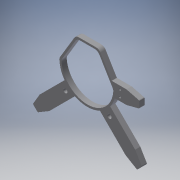
# Autodesk Inventor part: PearHeadbar
Saved by Autodesk Inventor 2016 (Build 200138000, 138)
## iProperties
Created: 2015-02-26
Part Number: PearHeadbar
Material: Generic
Document SubType Name: Modeling
Designer: ChurchlandLab
Density: 1 g/cm^3
Sheet Metal Rule: Default
Appearance: Default
Author: ChurchlandLab
Autodesk Inventor part; units mm, degrees
ref_plane "YZ Plane" through (0, 0, 0) normal (1, 0, 0) x (0, 1, 0)
ref_plane "XZ Plane" through (0, 0, 0) normal (0, 1, 0) x (-1, 0, 0)
ref_plane "XY Plane" through (0, 0, 0) normal (0, 0, 1) x (1, 0, 0)
sketch "Sketch1" plane through (0, 0, 0) normal (0, 0, 1) x (1, 0, 0)
  line L0 (0, 9.6891) -> (0, -0.0008) construction
  arc A0 (-6.35, -0.0008) -> (6.35, -0.0008) centre (0, -0.0008) ccw
  line L1 (9.3613, -12.4169) -> (3.0751, -6.1307)
  line L2 (5.5891, -3.975) -> (11.6964, -10.0822)
  line L3 (9.3613, -12.4169) -> (12.1811, -14.0872)
  line L4 (12.1811, -14.0872) -> (13.3665, -12.9018)
  line L5 (13.3665, -12.9018) -> (11.6964, -10.0822)
  line L6 (19.3321, -0.0008) -> (-6.0679, -0.0008) construction
  arc A1 (-3.0752, -6.1307) -> (3.0751, -6.1307) centre (0, -0.0008) ccw
  arc A2 (0.9808, -6.7883) -> (3.0751, -6.1307) centre (0, -0.0008) ccw
  arc A3 (-6.8102, -0.809) -> (-5.5892, -3.975) centre (0, -0.0008) ccw
  arc A4 (5.5891, -3.975) -> (6.6548, -1.6576) centre (0, -0.0008) ccw
  arc A5 (5.5891, -3.975) -> (6.6548, -1.6576) centre (0, -0.0008) ccw
  line L7 (5.5891, -3.975) -> (21.5654, -3.975) construction
  line L8 (-9.3614, -12.4169) -> (-3.0752, -6.1307)
  line L9 (-5.5892, -3.975) -> (-11.6964, -10.0822)
  line L10 (-9.3614, -12.4169) -> (-12.1812, -14.0872)
  line L11 (-12.1812, -14.0872) -> (-13.3666, -12.9018)
  line L12 (-13.3666, -12.9018) -> (-11.6964, -10.0822)
  line L13 (9.5758, 1.6559) -> (12.7495, 0.8434)
  line L14 (6.6548, 1.6559) -> (9.5758, 1.6559)
  line L15 (9.5758, -1.6576) -> (12.7495, -0.8451)
  line L16 (6.6548, -1.6576) -> (9.5758, -1.6576)
  circle A6 centre (7.9375, -0.7946) radius 0.254
  circle A7 centre (7.9375, 0.7929) radius 0.254
  circle A8 centre (-5.4113, -6.1454) radius 0.508
  line L17 (12.7495, 0.8434) -> (12.7495, -0.8451)
  circle A9 centre (5.4113, -6.1454) radius 0.508
  line L18 (-2.5412, 6.3492) -> (2.5411, 6.3492)
  line L19 (2.5411, 6.3492) -> (6.35, -0.0008)
  line L20 (5.9486, 1.6559) -> (6.6548, 1.6559)
  line L21 (5.9486, 1.6559) -> (2.8288, 6.8572)
  line L22 (2.8288, 6.8572) -> (-2.8289, 6.8572)
  arc A10 (-6.8565, 0.1423) -> (-5.5892, -3.975) centre (0, -0.0008) ccw
  line L23 (0, 6.3492) -> (-2.5412, 6.3492)
  line L24 (-2.5412, 6.3492) -> (-6.35, -0.0008)
  line L25 (-6.8565, 0.1423) -> (-2.8289, 6.8572)
  line L26 (-2.8289, 6.8572) -> (0, 6.8572)
  point P0 (13.4194, -0.6736)
  point P1 (13.4673, -0.0008)
  point P2 (0, 7.922)
  dimension "GapSize" = 3.048
  dimension "d35" = 12.7
  dimension "d72" = 8.89
  dimension "d73" = 3.2774
  dimension "d77" = 194.36
  dimension "d78" = 1.6764
  dimension "d115" = 90
  dimension "d127" = 0.508
  dimension "d128" = 165.64
  dimension "d154" = 3.302
  dimension "d160" = 3.276
  dimension "d166" = 0.508
  dimension "d168" = 7.9375
  dimension "d169" = 0.863
  dimension "d176" = 1.016
  dimension "d182" = 3.3135
  dimension "d184" = 1.6885
  dimension "d191" = 2.921
  dimension "d234" = 24.3623
  dimension "d238" = 0.508
  dimension "d239" = 0.508
  dimension "d240" = 0.508
  dimension "d241" = 25.4
  dimension "d242" = 0.508
  constraints: 54 end point, 15 point on circle, 13 symmetric about line, 11 centre point, 6 point on line, 4 perpendicular, 2 horizontal, 2 midpoint, 1 coincident, 1 parallel, 1 tangent, 1 vertical, 2 other
  measures "d35" diameter of A0
  measures "d72" distance of L1.end L1.start
  measures "d73" distance of L1.start L3.end
  measures "d78" distance of L3.end L4.end
  measures "d115" angle of L0 L6
  measures "d127" radial gap between concentric circles of A0 A1
  measures "d128" angle of L5 L2
  measures "d154" distance between parallel lines of L1 L2
  measures "d160" distance of L13.start L13.end
  measures "d166" diameter of A6
  measures "d168" horizontal distance of L0.end A6.centre
  measures "d169" distance from line of L16 A6.centre
  measures "d176" diameter of A8
  measures "d182" distance of L16.start L14.start
  measures "d184" distance of L13.end L15.end
  measures "d191" distance of L14.start L13.start
  measures "d234" distance of L10.end L3.end
  measures "d238" distance between parallel lines of L21 L19
  measures "d239" distance between parallel lines of L22 L18
  measures "d240" distance between parallel lines of L25 L24
  measures "d241" distance of L6.start L6.end
  measures "d242" radial gap between concentric circles of A0 A10
extrude "Extrusion9" add sketch "Sketch1" along normal blind 1.27
fillet "Fillet67" radius 0.254 1 edges at (12.7495, 0.8434, 0.635)
fillet "Fillet68" radius 0.254 1 edges at (12.7495, -0.8451, 0.635)
fillet "Fillet69" radius 1.27 1 edges at (6.35, -0.0008, 0.635)
fillet "Fillet70" radius 1.27 1 edges at (2.8288, 6.8572, 0.635)
fillet "Fillet71" radius 1.27 1 edges at (-2.8289, 6.8572, 0.635)
fillet "Fillet72" radius 1.27 1 edges at (-6.8565, 0.1423, 0.635)
fillet "Fillet73" radius 1.27 1 edges at (-6.35, -0.0008, 0.635)
fillet "Fillet74" radius 1.27 1 edges at (2.5411, 6.3492, 0.635)
fillet "Fillet75" radius 1.27 1 edges at (-2.5412, 6.3492, 0.635)
fillet "Fillet76" radius 0.254 1 edges at (13.3665, -12.9018, 0.635)
fillet "Fillet77" radius 0.254 1 edges at (12.1811, -14.0872, 0.635)
fillet "Fillet78" radius 0.254 1 edges at (-12.1812, -14.0872, 0.635)
fillet "Fillet79" radius 0.254 1 edges at (-13.3666, -12.9018, 0.635)
equation "\"GapSize\" = Thickness"
equation "\"BendRadius\" = Thickness"
equation "\"BendReliefWidth\" = Thickness"
equation "\"BendReliefDepth\" = 0.5 * Thickness"
equation "\"CornerReliefSize\" = 4 * Thickness"
equation "\"MinimumRemnant\" = 2 * Thickness"
equation "\"TransitionRadius\" = BendRadius"
equation "\"JacobiRadiusSize\" = BendRadius"
equation "\"Thickness\" = 3.048"
body "Solid8"
